Autodesk Fusion 360 part; units mm, degrees
(part 6 of 6)
  spline S39 degree 5 poles (-10.607, 23.738) (-10.6081, 23.7269) (-10.6103, 23.7048) (-10.6136, 23.6717) (-10.6177, 23.6275) (-10.6227, 23.5724) (-10.6274, 23.5173) (-10.6319, 23.4622) (-10.6361, 23.4072) (-10.6401, 23.3523) (-10.6438, 23.2974) (-10.6473, 23.2426) (-10.6505, 23.1878) (-10.6534, 23.133) (-10.6561, 23.0784) (-10.6586, 23.0238) (-10.6607, 22.9692) (-10.6627, 22.9147) (-10.6643, 22.8603) (-10.6657, 22.8059) (-10.6668, 22.7516) (-10.6677, 22.6974) (-10.6683, 22.6432) (-10.6686, 22.5891) (-10.6686, 22.5351) (-10.6684, 22.4812) (-10.6679, 22.4273) (-10.6671, 22.3735) (-10.6661, 22.3198) (-10.6647, 22.2661) (-10.6631, 22.2126) (-10.6612, 22.1591) (-10.659, 22.1057) (-10.6565, 22.0524) (-10.6537, 21.9992) (-10.6506, 21.9461) (-10.6473, 21.893) (-10.6436, 21.8401) (-10.6396, 21.7872) (-10.6353, 21.7345) (-10.6307, 21.6818) (-10.6258, 21.6293) (-10.6205, 21.5768) (-10.615, 21.5245) (-10.6091, 21.4723) (-10.6028, 21.4202) (-10.5963, 21.3682) (-10.5894, 21.3163) (-10.5822, 21.2645) (-10.5746, 21.2129) (-10.5667, 21.1614) (-10.5583, 21.11) (-10.5496, 21.0588) (-10.5405, 21.0078) (-10.531, 20.9569) (-10.5211, 20.9061) (-10.5109, 20.8555) (-10.5003, 20.805) (-10.4893, 20.7546) (-10.4779, 20.7044) (-10.466, 20.6545) (-10.4535, 20.6048) (-10.4404, 20.5553) (-10.4266, 20.5061) (-10.4123, 20.4572) (-10.3976, 20.4084) (-10.3826, 20.3597) (-10.3673, 20.3113) (-10.3516, 20.263) (-10.335, 20.2151) (-10.3172, 20.1677) (-10.3015, 20.1305) (-10.2887, 20.103) (-10.2797, 20.0849) (-10.2751, 20.0759) knots -1 -1 -1 -1 -1 -1 -0.98571429 -0.97142857 -0.95714286 -0.94285714 -0.92857143 -0.91428571 -0.9 -0.88571429 -0.87142857 -0.85714286 -0.84285714 -0.82857143 -0.81428571 -0.8 -0.78571429 -0.77142857 -0.75714286 -0.74285714 -0.72857143 -0.71428571 -0.7 -0.68571429 -0.67142857 -0.65714286 -0.64285714 -0.62857143 -0.61428571 -0.6 -0.58571429 -0.57142857 -0.55714286 -0.54285714 -0.52857143 -0.51428571 -0.5 -0.48571429 -0.47142857 -0.45714286 -0.44285714 -0.42857143 -0.41428571 -0.4 -0.38571429 -0.37142857 -0.35714286 -0.34285714 -0.32857143 -0.31428571 -0.3 -0.28571429 -0.27142857 -0.25714286 -0.24285714 -0.22857143 -0.21428571 -0.2 -0.18571429 -0.17142857 -0.15714286 -0.14285714 -0.12857143 -0.11428571 -0.1 -0.08571429 -0.07142857 -0.05714286 -0.04285714 -0.02857143 -0.01428571 0 0 0 0 0 0
  line L43 (-10.2751, 20.0759) -> (-10.2631, 20.0524)
  arc A79 (-10.659, 18.7284) -> (-10.2631, 20.0524) centre (-11.1537, 19.5975) ccw
  arc A80 (-10.659, 18.7284) -> (-10.8898, 18.5952) centre (0, 0) ccw
  arc A81 (-12.2343, 18.9143) -> (-10.8898, 18.5952) centre (-11.3951, 19.4581) ccw
  line L44 (-12.2343, 18.9143) -> (-12.2487, 18.9365)
  spline S40 degree 5 poles (-12.2487, 18.9365) (-12.2542, 18.945) (-12.2654, 18.9618) (-12.2828, 18.9866) (-12.3072, 19.0188) (-12.3392, 19.0579) (-12.3725, 19.0962) (-12.4064, 19.134) (-12.4407, 19.1715) (-12.4754, 19.2088) (-12.5103, 19.2459) (-12.5455, 19.2828) (-12.5812, 19.3193) (-12.6175, 19.3554) (-12.6543, 19.3911) (-12.6916, 19.4264) (-12.7294, 19.4613) (-12.7675, 19.496) (-12.8059, 19.5304) (-12.8447, 19.5646) (-12.8837, 19.5985) (-12.923, 19.6322) (-12.9627, 19.6656) (-13.0027, 19.6988) (-13.043, 19.7317) (-13.0836, 19.7643) (-13.1245, 19.7967) (-13.1658, 19.8288) (-13.2072, 19.8607) (-13.249, 19.8924) (-13.291, 19.9239) (-13.3333, 19.9551) (-13.3758, 19.9861) (-13.4186, 20.0168) (-13.4616, 20.0474) (-13.5049, 20.0777) (-13.5485, 20.1078) (-13.5923, 20.1376) (-13.6363, 20.1673) (-13.6805, 20.1968) (-13.725, 20.226) (-13.7697, 20.255) (-13.8146, 20.2838) (-13.8597, 20.3124) (-13.9051, 20.3408) (-13.9507, 20.369) (-13.9965, 20.397) (-14.0425, 20.4248) (-14.0887, 20.4523) (-14.1351, 20.4797) (-14.1817, 20.5069) (-14.2285, 20.5339) (-14.2755, 20.5606) (-14.3227, 20.5872) (-14.3701, 20.6136) (-14.4177, 20.6397) (-14.4654, 20.6657) (-14.5134, 20.6915) (-14.5615, 20.7171) (-14.6099, 20.7425) (-14.6584, 20.7676) (-14.7071, 20.7926) (-14.756, 20.8175) (-14.805, 20.8421) (-14.8542, 20.8665) (-14.9036, 20.8907) (-14.9532, 20.9147) (-15.0029, 20.9386) (-15.0529, 20.9622) (-15.1029, 20.9857) (-15.1532, 21.009) (-15.1935, 21.0275) (-15.2238, 21.0412) (-15.2441, 21.0504) (-15.2542, 21.0549) knots 0 0 0 0 0 0 0.01428571 0.02857143 0.04285714 0.05714286 0.07142857 0.08571429 0.1 0.11428571 0.12857143 0.14285714 0.15714286 0.17142857 0.18571429 0.2 0.21428571 0.22857143 0.24285714 0.25714286 0.27142857 0.28571429 0.3 0.31428571 0.32857143 0.34285714 0.35714286 0.37142857 0.38571429 0.4 0.41428571 0.42857143 0.44285714 0.45714286 0.47142857 0.48571429 0.5 0.51428571 0.52857143 0.54285714 0.55714286 0.57142857 0.58571429 0.6 0.61428571 0.62857143 0.64285714 0.65714286 0.67142857 0.68571429 0.7 0.71428571 0.72857143 0.74285714 0.75714286 0.77142857 0.78571429 0.8 0.81428571 0.82857143 0.84285714 0.85714286 0.87142857 0.88571429 0.9 0.91428571 0.92857143 0.94285714 0.95714286 0.97142857 0.98571429 1 1 1 1 1 1
  arc A82 (-15.2542, 21.0549) -> (-16.3894, 20.1838) centre (0, 0) ccw
  spline S41 degree 5 poles (-16.3894, 20.1838) (-16.3876, 20.1729) (-16.384, 20.1509) (-16.3786, 20.1181) (-16.3712, 20.0744) (-16.3617, 20.0198) (-16.352, 19.9654) (-16.3421, 19.911) (-16.3319, 19.8568) (-16.3215, 19.8027) (-16.3109, 19.7487) (-16.3001, 19.6949) (-16.289, 19.6411) (-16.2777, 19.5875) (-16.2661, 19.534) (-16.2544, 19.4806) (-16.2423, 19.4273) (-16.2301, 19.3742) (-16.2176, 19.3212) (-16.2049, 19.2683) (-16.1919, 19.2156) (-16.1787, 19.163) (-16.1653, 19.1105) (-16.1516, 19.0582) (-16.1376, 19.006) (-16.1235, 18.954) (-16.109, 18.9021) (-16.0944, 18.8503) (-16.0794, 18.7987) (-16.0643, 18.7472) (-16.0488, 18.6959) (-16.0331, 18.6447) (-16.0172, 18.5937) (-16.001, 18.5429) (-15.9845, 18.4922) (-15.9678, 18.4417) (-15.9508, 18.3913) (-15.9335, 18.3411) (-15.916, 18.2911) (-15.8982, 18.2413) (-15.8801, 18.1916) (-15.8618, 18.1421) (-15.8431, 18.0928) (-15.8242, 18.0437) (-15.805, 17.9948) (-15.7855, 17.9461) (-15.7657, 17.8976) (-15.7456, 17.8492) (-15.7253, 17.8011) (-15.7046, 17.7532) (-15.6836, 17.7055) (-15.6622, 17.658) (-15.6406, 17.6108) (-15.6185, 17.5639) (-15.5962, 17.5172) (-15.5735, 17.4707) (-15.5505, 17.4244) (-15.5272, 17.3784) (-15.5036, 17.3326) (-15.4796, 17.2871) (-15.4552, 17.2419) (-15.4302, 17.1971) (-15.4048, 17.1527) (-15.3787, 17.1088) (-15.3523, 17.0652) (-15.3254, 17.0219) (-15.2983, 16.9788) (-15.271, 16.9359) (-15.2433, 16.8933) (-15.2149, 16.8513) (-15.1854, 16.8103) (-15.1606, 16.7784) (-15.1412, 16.7551) (-15.1278, 16.74) (-15.121, 16.7325) knots -1 -1 -1 -1 -1 -1 -0.98571429 -0.97142857 -0.95714286 -0.94285714 -0.92857143 -0.91428571 -0.9 -0.88571429 -0.87142857 -0.85714286 -0.84285714 -0.82857143 -0.81428571 -0.8 -0.78571429 -0.77142857 -0.75714286 -0.74285714 -0.72857143 -0.71428571 -0.7 -0.68571429 -0.67142857 -0.65714286 -0.64285714 -0.62857143 -0.61428571 -0.6 -0.58571429 -0.57142857 -0.55714286 -0.54285714 -0.52857143 -0.51428571 -0.5 -0.48571429 -0.47142857 -0.45714286 -0.44285714 -0.42857143 -0.41428571 -0.4 -0.38571429 -0.37142857 -0.35714286 -0.34285714 -0.32857143 -0.31428571 -0.3 -0.28571429 -0.27142857 -0.25714286 -0.24285714 -0.22857143 -0.21428571 -0.2 -0.18571429 -0.17142857 -0.15714286 -0.14285714 -0.12857143 -0.11428571 -0.1 -0.08571429 -0.07142857 -0.05714286 -0.04285714 -0.02857143 -0.01428571 0 0 0 0 0 0
  line L45 (-15.121, 16.7325) -> (-15.1034, 16.7129)
  arc A83 (-15.1431, 15.3315) -> (-15.1034, 16.7129) centre (-15.8458, 16.043) ccw
  arc A84 (-15.1431, 15.3315) -> (-15.3315, 15.1431) centre (0, 0) ccw
  arc A85 (-16.7129, 15.1034) -> (-15.3315, 15.1431) centre (-16.043, 15.8458) ccw
  line L46 (-16.7129, 15.1034) -> (-16.7325, 15.121)
  spline S42 degree 5 poles (-16.7325, 15.121) (-16.74, 15.1278) (-16.7551, 15.1412) (-16.7784, 15.1606) (-16.8103, 15.1854) (-16.8513, 15.2149) (-16.8933, 15.2433) (-16.9359, 15.271) (-16.9788, 15.2983) (-17.0219, 15.3254) (-17.0652, 15.3523) (-17.1088, 15.3787) (-17.1527, 15.4048) (-17.1971, 15.4302) (-17.2419, 15.4552) (-17.2871, 15.4796) (-17.3326, 15.5036) (-17.3784, 15.5272) (-17.4244, 15.5505) (-17.4707, 15.5735) (-17.5172, 15.5962) (-17.5639, 15.6185) (-17.6108, 15.6406) (-17.658, 15.6622) (-17.7055, 15.6836) (-17.7532, 15.7046) (-17.8011, 15.7253) (-17.8492, 15.7456) (-17.8976, 15.7657) (-17.9461, 15.7855) (-17.9948, 15.805) (-18.0437, 15.8242) (-18.0928, 15.8431) (-18.1421, 15.8618) (-18.1916, 15.8801) (-18.2413, 15.8982) (-18.2911, 15.916) (-18.3411, 15.9335) (-18.3913, 15.9508) (-18.4417, 15.9678) (-18.4922, 15.9845) (-18.5429, 16.001) (-18.5937, 16.0172) (-18.6447, 16.0331) (-18.6959, 16.0488) (-18.7472, 16.0643) (-18.7987, 16.0794) (-18.8503, 16.0944) (-18.9021, 16.109) (-18.954, 16.1235) (-19.006, 16.1376) (-19.0582, 16.1516) (-19.1105, 16.1653) (-19.163, 16.1787) (-19.2156, 16.1919) (-19.2683, 16.2049) (-19.3212, 16.2176) (-19.3742, 16.2301) (-19.4273, 16.2423) (-19.4806, 16.2544) (-19.534, 16.2661) (-19.5875, 16.2777) (-19.6411, 16.289) (-19.6949, 16.3001) (-19.7487, 16.3109) (-19.8027, 16.3215) (-19.8568, 16.3319) (-19.911, 16.3421) (-19.9654, 16.352) (-20.0198, 16.3617) (-20.0744, 16.3712) (-20.1181, 16.3786) (-20.1509, 16.384) (-20.1729, 16.3876) (-20.1838, 16.3894) knots 0 0 0 0 0 0 0.01428571 0.02857143 0.04285714 0.05714286 0.07142857 0.08571429 0.1 0.11428571 0.12857143 0.14285714 0.15714286 0.17142857 0.18571429 0.2 0.21428571 0.22857143 0.24285714 0.25714286 0.27142857 0.28571429 0.3 0.31428571 0.32857143 0.34285714 0.35714286 0.37142857 0.38571429 0.4 0.41428571 0.42857143 0.44285714 0.45714286 0.47142857 0.48571429 0.5 0.51428571 0.52857143 0.54285714 0.55714286 0.57142857 0.58571429 0.6 0.61428571 0.62857143 0.64285714 0.65714286 0.67142857 0.68571429 0.7 0.71428571 0.72857143 0.74285714 0.75714286 0.77142857 0.78571429 0.8 0.81428571 0.82857143 0.84285714 0.85714286 0.87142857 0.88571429 0.9 0.91428571 0.92857143 0.94285714 0.95714286 0.97142857 0.98571429 1 1 1 1 1 1
  arc A86 (-20.1838, 16.3894) -> (-21.0549, 15.2542) centre (0, 0) ccw
  spline S43 degree 5 poles (-21.0549, 15.2542) (-21.0504, 15.2441) (-21.0412, 15.2238) (-21.0275, 15.1935) (-21.009, 15.1532) (-20.9857, 15.1029) (-20.9622, 15.0529) (-20.9386, 15.0029) (-20.9147, 14.9532) (-20.8907, 14.9036) (-20.8665, 14.8542) (-20.8421, 14.805) (-20.8175, 14.756) (-20.7926, 14.7071) (-20.7676, 14.6584) (-20.7425, 14.6099) (-20.7171, 14.5615) (-20.6915, 14.5134) (-20.6657, 14.4654) (-20.6397, 14.4177) (-20.6136, 14.3701) (-20.5872, 14.3227) (-20.5606, 14.2755) (-20.5339, 14.2285) (-20.5069, 14.1817) (-20.4797, 14.1351) (-20.4523, 14.0887) (-20.4248, 14.0425) (-20.397, 13.9965) (-20.369, 13.9507) (-20.3408, 13.9051) (-20.3124, 13.8597) (-20.2838, 13.8146) (-20.255, 13.7697) (-20.226, 13.725) (-20.1968, 13.6805) (-20.1673, 13.6363) (-20.1376, 13.5923) (-20.1078, 13.5485) (-20.0777, 13.5049) (-20.0474, 13.4616) (-20.0168, 13.4186) (-19.9861, 13.3758) (-19.9551, 13.3333) (-19.9239, 13.291) (-19.8924, 13.249) (-19.8607, 13.2072) (-19.8288, 13.1658) (-19.7967, 13.1245) (-19.7643, 13.0836) (-19.7317, 13.043) (-19.6988, 13.0027) (-19.6656, 12.9627) (-19.6322, 12.923) (-19.5985, 12.8837) (-19.5646, 12.8447) (-19.5304, 12.8059) (-19.496, 12.7675) (-19.4613, 12.7294) (-19.4264, 12.6916) (-19.3911, 12.6543) (-19.3554, 12.6175) (-19.3193, 12.5812) (-19.2828, 12.5455) (-19.2459, 12.5103) (-19.2088, 12.4754) (-19.1715, 12.4407) (-19.134, 12.4064) (-19.0962, 12.3725) (-19.0579, 12.3392) (-19.0188, 12.3072) (-18.9866, 12.2828) (-18.9618, 12.2654) (-18.945, 12.2542) (-18.9365, 12.2487) knots -1 -1 -1 -1 -1 -1 -0.98571429 -0.97142857 -0.95714286 -0.94285714 -0.92857143 -0.91428571 -0.9 -0.88571429 -0.87142857 -0.85714286 -0.84285714 -0.82857143 -0.81428571 -0.8 -0.78571429 -0.77142857 -0.75714286 -0.74285714 -0.72857143 -0.71428571 -0.7 -0.68571429 -0.67142857 -0.65714286 -0.64285714 -0.62857143 -0.61428571 -0.6 -0.58571429 -0.57142857 -0.55714286 -0.54285714 -0.52857143 -0.51428571 -0.5 -0.48571429 -0.47142857 -0.45714286 -0.44285714 -0.42857143 -0.41428571 -0.4 -0.38571429 -0.37142857 -0.35714286 -0.34285714 -0.32857143 -0.31428571 -0.3 -0.28571429 -0.27142857 -0.25714286 -0.24285714 -0.22857143 -0.21428571 -0.2 -0.18571429 -0.17142857 -0.15714286 -0.14285714 -0.12857143 -0.11428571 -0.1 -0.08571429 -0.07142857 -0.05714286 -0.04285714 -0.02857143 -0.01428571 0 0 0 0 0 0
  line L47 (-18.9365, 12.2487) -> (-18.9143, 12.2343)
  arc A87 (-18.5952, 10.8898) -> (-18.9143, 12.2343) centre (-19.4581, 11.3951) ccw
  arc A88 (-18.5952, 10.8898) -> (-18.7284, 10.659) centre (0, 0) ccw
  arc A89 (-20.0524, 10.2631) -> (-18.7284, 10.659) centre (-19.5975, 11.1537) ccw
  line L48 (-20.0524, 10.2631) -> (-20.0759, 10.2751)
  spline S44 degree 5 poles (-20.0759, 10.2751) (-20.0849, 10.2797) (-20.103, 10.2887) (-20.1305, 10.3015) (-20.1677, 10.3172) (-20.2151, 10.335) (-20.263, 10.3516) (-20.3113, 10.3673) (-20.3597, 10.3826) (-20.4084, 10.3976) (-20.4572, 10.4123) (-20.5061, 10.4266) (-20.5553, 10.4404) (-20.6048, 10.4535) (-20.6545, 10.466) (-20.7044, 10.4779) (-20.7546, 10.4893) (-20.805, 10.5003) (-20.8555, 10.5109) (-20.9061, 10.5211) (-20.9569, 10.531) (-21.0078, 10.5405) (-21.0588, 10.5496) (-21.11, 10.5583) (-21.1614, 10.5667) (-21.2129, 10.5746) (-21.2645, 10.5822) (-21.3163, 10.5894) (-21.3682, 10.5963) (-21.4202, 10.6028) (-21.4723, 10.6091) (-21.5245, 10.615) (-21.5768, 10.6205) (-21.6293, 10.6258) (-21.6818, 10.6307) (-21.7345, 10.6353) (-21.7872, 10.6396) (-21.8401, 10.6436) (-21.893, 10.6473) (-21.9461, 10.6506) (-21.9992, 10.6537) (-22.0524, 10.6565) (-22.1057, 10.659) (-22.1591, 10.6612) (-22.2126, 10.6631) (-22.2661, 10.6647) (-22.3198, 10.6661) (-22.3735, 10.6671) (-22.4273, 10.6679) (-22.4812, 10.6684) (-22.5351, 10.6686) (-22.5891, 10.6686) (-22.6432, 10.6683) (-22.6974, 10.6677) (-22.7516, 10.6668) (-22.8059, 10.6657) (-22.8603, 10.6643) (-22.9147, 10.6627) (-22.9692, 10.6607) (-23.0238, 10.6586) (-23.0784, 10.6561) (-23.133, 10.6534) (-23.1878, 10.6505) (-23.2426, 10.6473) (-23.2974, 10.6438) (-23.3523, 10.6401) (-23.4072, 10.6361) (-23.4622, 10.6319) (-23.5173, 10.6274) (-23.5724, 10.6227) (-23.6275, 10.6177) (-23.6717, 10.6136) (-23.7048, 10.6103) (-23.7269, 10.6081) (-23.738, 10.607) knots 0 0 0 0 0 0 0.01428571 0.02857143 0.04285714 0.05714286 0.07142857 0.08571429 0.1 0.11428571 0.12857143 0.14285714 0.15714286 0.17142857 0.18571429 0.2 0.21428571 0.22857143 0.24285714 0.25714286 0.27142857 0.28571429 0.3 0.31428571 0.32857143 0.34285714 0.35714286 0.37142857 0.38571429 0.4 0.41428571 0.42857143 0.44285714 0.45714286 0.47142857 0.48571429 0.5 0.51428571 0.52857143 0.54285714 0.55714286 0.57142857 0.58571429 0.6 0.61428571 0.62857143 0.64285714 0.65714286 0.67142857 0.68571429 0.7 0.71428571 0.72857143 0.74285714 0.75714286 0.77142857 0.78571429 0.8 0.81428571 0.82857143 0.84285714 0.85714286 0.87142857 0.88571429 0.9 0.91428571 0.92857143 0.94285714 0.95714286 0.97142857 0.98571429 1 1 1 1 1 1
  arc A90 (-23.738, 10.607) -> (-24.2856, 9.285) centre (0, 0) ccw
  spline S45 degree 5 poles (-24.2856, 9.285) (-24.2785, 9.2764) (-24.2645, 9.2592) (-24.2433, 9.2335) (-24.2151, 9.1993) (-24.1796, 9.1568) (-24.1439, 9.1145) (-24.1082, 9.0724) (-24.0723, 9.0306) (-24.0362, 8.9889) (-24, 8.9474) (-23.9637, 8.9062) (-23.9272, 8.8652) (-23.8906, 8.8244) (-23.8539, 8.7839) (-23.817, 8.7435) (-23.78, 8.7034) (-23.7428, 8.6635) (-23.7055, 8.6239) (-23.668, 8.5844) (-23.6304, 8.5452) (-23.5927, 8.5063) (-23.5548, 8.4676) (-23.5168, 8.4291) (-23.4786, 8.3909) (-23.4403, 8.3529) (-23.4019, 8.3151) (-23.3633, 8.2777) (-23.3245, 8.2404) (-23.2857, 8.2034) (-23.2466, 8.1667) (-23.2075, 8.1302) (-23.1682, 8.094) (-23.1287, 8.0581) (-23.0891, 8.0225) (-23.0493, 7.9871) (-23.0095, 7.9519) (-22.9694, 7.9171) (-22.9292, 7.8826) (-22.8889, 7.8483) (-22.8484, 7.8143) (-22.8078, 7.7806) (-22.767, 7.7473) (-22.726, 7.7142) (-22.6849, 7.6815) (-22.6437, 7.649) (-22.6023, 7.6169) (-22.5607, 7.5851) (-22.519, 7.5536) (-22.4772, 7.5224) (-22.4351, 7.4916) (-22.3929, 7.4612) (-22.3505, 7.4311) (-22.308, 7.4015) (-22.2653, 7.3722) (-22.2224, 7.3433) (-22.1793, 7.3147) (-22.1361, 7.2865) (-22.0928, 7.2587) (-22.0493, 7.2312) (-22.0055, 7.2043) (-21.9615, 7.178) (-21.9173, 7.1523) (-21.8728, 7.1273) (-21.828, 7.1028) (-21.7832, 7.0787) (-21.7381, 7.0549) (-21.693, 7.0314) (-21.6478, 7.0084) (-21.6022, 6.9862) (-21.5561, 6.9654) (-21.5187, 6.9502) (-21.4902, 6.9398) (-21.471, 6.9333) (-21.4614, 6.9302) knots -1 -1 -1 -1 -1 -1 -0.98571429 -0.97142857 -0.95714286 -0.94285714 -0.92857143 -0.91428571 -0.9 -0.88571429 -0.87142857 -0.85714286 -0.84285714 -0.82857143 -0.81428571 -0.8 -0.78571429 -0.77142857 -0.75714286 -0.74285714 -0.72857143 -0.71428571 -0.7 -0.68571429 -0.67142857 -0.65714286 -0.64285714 -0.62857143 -0.61428571 -0.6 -0.58571429 -0.57142857 -0.55714286 -0.54285714 -0.52857143 -0.51428571 -0.5 -0.48571429 -0.47142857 -0.45714286 -0.44285714 -0.42857143 -0.41428571 -0.4 -0.38571429 -0.37142857 -0.35714286 -0.34285714 -0.32857143 -0.31428571 -0.3 -0.28571429 -0.27142857 -0.25714286 -0.24285714 -0.22857143 -0.21428571 -0.2 -0.18571429 -0.17142857 -0.15714286 -0.14285714 -0.12857143 -0.11428571 -0.1 -0.08571429 -0.07142857 -0.05714286 -0.04285714 -0.02857143 -0.01428571 0 0 0 0 0 0
  line L49 (-21.4614, 6.9302) -> (-21.4363, 6.9221)
  arc A91 (-20.78, 5.7059) -> (-21.4363, 6.9221) centre (-21.7444, 5.9707) ccw
  arc A92 (-20.78, 5.7059) -> (-20.849, 5.4485) centre (0, 0) ccw
  arc A93 (-22.0254, 4.7235) -> (-20.849, 5.4485) centre (-21.8165, 5.7014) ccw
  line L50 (-22.0254, 4.7235) -> (-22.0512, 4.729)
  spline S46 degree 5 poles (-22.0512, 4.729) (-22.0611, 4.7311) (-22.081, 4.7351) (-22.1108, 4.7403) (-22.1508, 4.7458) (-22.2011, 4.7508) (-22.2517, 4.7544) (-22.3024, 4.7571) (-22.3532, 4.7594) (-22.4041, 4.7613) (-22.455, 4.7629) (-22.506, 4.764) (-22.5571, 4.7645) (-22.6082, 4.7644) (-22.6595, 4.7636) (-22.7108, 4.7622) (-22.7623, 4.7602) (-22.8137, 4.7578) (-22.8652, 4.7549) (-22.9168, 4.7517) (-22.9684, 4.7481) (-23.02, 4.7441) (-23.0717, 4.7397) (-23.1234, 4.7349) (-23.1752, 4.7296) (-23.227, 4.724) (-23.2788, 4.7179) (-23.3307, 4.7115) (-23.3826, 4.7047) (-23.4345, 4.6976) (-23.4865, 4.6901) (-23.5384, 4.6823) (-23.5904, 4.6742) (-23.6424, 4.6656) (-23.6945, 4.6568) (-23.7465, 4.6476) (-23.7986, 4.6381) (-23.8506, 4.6283) (-23.9027, 4.6181) (-23.9548, 4.6077) (-24.007, 4.5969) (-24.0591, 4.5858) (-24.1112, 4.5744) (-24.1634, 4.5627) (-24.2155, 4.5507) (-24.2677, 4.5384) (-24.3198, 4.5259) (-24.372, 4.513) (-24.4242, 4.4998) (-24.4763, 4.4863) (-24.5285, 4.4726) (-24.5807, 4.4586) (-24.6328, 4.4443) (-24.685, 4.4297) (-24.7372, 4.4148) (-24.7893, 4.3997) (-24.8415, 4.3843) (-24.8936, 4.3686) (-24.9458, 4.3526) (-24.9979, 4.3364) (-25.05, 4.3199) (-25.1021, 4.3031) (-25.1542, 4.2861) (-25.2063, 4.2688) (-25.2584, 4.2513) (-25.3104, 4.2335) (-25.3625, 4.2154) (-25.4145, 4.1971) (-25.4665, 4.1786) (-25.5185, 4.1598) (-25.5705, 4.1407) (-25.6121, 4.1252) (-25.6433, 4.1135) (-25.664, 4.1057) (-25.6744, 4.1017) knots 0 0 0 0 0 0 0.01428571 0.02857143 0.04285714 0.05714286 0.07142857 0.08571429 0.1 0.11428571 0.12857143 0.14285714 0.15714286 0.17142857 0.18571429 0.2 0.21428571 0.22857143 0.24285714 0.25714286 0.27142857 0.28571429 0.3 0.31428571 0.32857143 0.34285714 0.35714286 0.37142857 0.38571429 0.4 0.41428571 0.42857143 0.44285714 0.45714286 0.47142857 0.48571429 0.5 0.51428571 0.52857143 0.54285714 0.55714286 0.57142857 0.58571429 0.6 0.61428571 0.62857143 0.64285714 0.65714286 0.67142857 0.68571429 0.7 0.71428571 0.72857143 0.74285714 0.75714286 0.77142857 0.78571429 0.8 0.81428571 0.82857143 0.84285714 0.85714286 0.87142857 0.88571429 0.9 0.91428571 0.92857143 0.94285714 0.95714286 0.97142857 0.98571429 1 1 1 1 1 1
  arc A94 (-25.6744, 4.1017) -> (-25.8612, 2.6831) centre (0, 0) ccw
  spline S47 degree 5 poles (-25.8612, 2.6831) (-25.8522, 2.6766) (-25.8341, 2.6636) (-25.8071, 2.6442) (-25.7709, 2.6185) (-25.7256, 2.5867) (-25.6803, 2.555) (-25.6348, 2.5236) (-25.5893, 2.4925) (-25.5437, 2.4616) (-25.498, 2.4309) (-25.4523, 2.4005) (-25.4064, 2.3703) (-25.3605, 2.3404) (-25.3145, 2.3107) (-25.2684, 2.2813) (-25.2223, 2.2521) (-25.1761, 2.2232) (-25.1297, 2.1946) (-25.0834, 2.1662) (-25.0369, 2.1381) (-24.9904, 2.1102) (-24.9438, 2.0826) (-24.8971, 2.0553) (-24.8503, 2.0282) (-24.8035, 2.0015) (-24.7566, 1.975) (-24.7096, 1.9487) (-24.6625, 1.9228) (-24.6154, 1.8971) (-24.5682, 1.8718) (-24.521, 1.8467) (-24.4736, 1.8219) (-24.4262, 1.7974) (-24.3787, 1.7732) (-24.3312, 1.7493) (-24.2835, 1.7257) (-24.2358, 1.7024) (-24.1881, 1.6794) (-24.1403, 1.6568) (-24.0924, 1.6344) (-24.0444, 1.6124) (-23.9963, 1.5908) (-23.9482, 1.5694) (-23.9001, 1.5484) (-23.8518, 1.5278) (-23.8035, 1.5075) (-23.7551, 1.4875) (-23.7067, 1.4678) (-23.6582, 1.4486) (-23.6096, 1.4297) (-23.561, 1.4112) (-23.5123, 1.3932) (-23.4635, 1.3756) (-23.4147, 1.3583) (-23.3658, 1.3415) (-23.3168, 1.3251) (-23.2678, 1.309) (-23.2187, 1.2933) (-23.1695, 1.2781) (-23.1203, 1.2634) (-23.071, 1.2494) (-23.0216, 1.236) (-22.9721, 1.2233) (-22.9226, 1.2112) (-22.873, 1.1996) (-22.8234, 1.1882) (-22.7737, 1.1773) (-22.724, 1.1668) (-22.6743, 1.1571) (-22.6244, 1.1489) (-22.5843, 1.1439) (-22.5541, 1.1413) (-22.5339, 1.14) (-22.5238, 1.1394) knots -1 -1 -1 -1 -1 -1 -0.98571429 -0.97142857 -0.95714286 -0.94285714 -0.92857143 -0.91428571 -0.9 -0.88571429 -0.87142857 -0.85714286 -0.84285714 -0.82857143 -0.81428571 -0.8 -0.78571429 -0.77142857 -0.75714286 -0.74285714 -0.72857143 -0.71428571 -0.7 -0.68571429 -0.67142857 -0.65714286 -0.64285714 -0.62857143 -0.61428571 -0.6 -0.58571429 -0.57142857 -0.55714286 -0.54285714 -0.52857143 -0.51428571 -0.5 -0.48571429 -0.47142857 -0.45714286 -0.44285714 -0.42857143 -0.41428571 -0.4 -0.38571429 -0.37142857 -0.35714286 -0.34285714 -0.32857143 -0.31428571 -0.3 -0.28571429 -0.27142857 -0.25714286 -0.24285714 -0.22857143 -0.21428571 -0.2 -0.18571429 -0.17142857 -0.15714286 -0.14285714 -0.12857143 -0.11428571 -0.1 -0.08571429 -0.07142857 -0.05714286 -0.04285714 -0.02857143 -0.01428571 0 0 0 0 0 0
  line L51 (-22.5238, 1.1394) -> (-22.4975, 1.1381)
  arc A95 (-21.5488, 0.1332) -> (-22.4975, 1.1381) centre (-22.5488, 0.1394) ccw
  circle A96 centre (0, 0) radius 6.35
  line L52 (-70, 15) -> (-24.9077, -25.8612)
  constraint coincident L1 L52.start
  constraint coincident L2 L52.end
sketch "スケッチ2 (4)" plane through (0, 0, 0) normal (0, 0, 1) x (-1, 0, 0)
  line L0 (80, 29.8124) -> (-70, 29.8124)
  line L1 (-70, 29.8124) -> (-70, -25.8612)
  line L2 (-70, -25.8612) -> (80, -25.8612)
  line L3 (80, -25.8612) -> (80, 29.8124)
sketch "スケッチ3 (3)" plane through (0, 0, -2) normal (0, 0, -1) x (1, 0, 0)
  line L0 (-80, -25.8612) -> (70, -25.8612)
  line L1 (70, -25.8612) -> (70, 29.8124)
  line L2 (70, 29.8124) -> (-80, 29.8124)
  line L3 (-80, 29.8124) -> (-80, -25.8612)
  circle A0 centre (0, 0) radius 16
  dimension "d32" = 32
  constraint coincident A0.centre origin
  measures "d32" diameter of A0
sketch "スケッチ4" plane through (0, 0, -2) normal (0, 0, -1) x (1, 0, 0)
  line L0 (-80, -25.8612) -> (70, -25.8612)
  line L1 (70, -25.8612) -> (70, 29.8124)
  line L2 (70, 29.8124) -> (-80, 29.8124)
  line L3 (-80, 29.8124) -> (-80, -25.8612)
  circle A0 centre (0, 0) radius 16
  circle A1 centre (0, 0) radius 6.2
  dimension "d35" = 12.4
  constraint coincident A0.centre A1.centre
  measures "d35" diameter of A1
extrude "押し出し3" cut sketch "スケッチ3 (3)" against normal blind 1 contours A0 bodies 24 in component "Base1"
extrude "押し出し4" cut sketch "スケッチ4" against normal blind 17 contours A1 bodies 24 in component "Base1"
sketch "スケッチ5" plane through (0, 0, -1) normal (0, 0, -1) x (1, 0, 0)
  circle A0 centre (0, 0) radius 6.2
  circle A1 centre (0, 0) radius 16
  circle A2 centre (0, 0) radius 6.35
  circle A3 centre (0, 0) radius 16
  line L0 (0, -25.8612) -> (0, 29.8124)
  circle A4 centre (0, 0) radius 6
  dimension "d38" = 12
  constraint coincident A0.centre A1.centre
  measures "d38" diameter of A4
extrude "押し出し1'''" add sketch "スケッチ5" against normal blind 15 separate body contours L0 A4 | L0 A4 makes body 25
sketch "スケッチ6" plane through (0, 0, -1) normal (0, 0, -1) x (1, 0, 0)
  circle A0 centre (0, 0) radius 6
  circle A1 centre (0, 0) radius 15.65
  dimension "d43" = 31.3
  constraint concentric A0 A1
  measures "d43" diameter of A1
extrude "押し出し2'''" add sketch "スケッチ5" sketch "スケッチ6" along normal blind 1 contours L0 A4 | L0 A4 of sketch 2 bodies 25
component "Spur Gear (24 teeth)" placed x (1, 0, 0) y (0, 1, 0) z (0, 0, 1) at (0, 0, 0)
component "Rack" placed x (1, 0, 0) y (0, 1, 0) z (0, 0, 1) at (0, 0, 0)
component "Base1" placed x (1, 0, 0) y (0, 1, 0) z (0, 0, 1) at (0, 0, 0)
equation "d12 = ( ( 360 / 24 ) / 2 ) * 1 deg"
equation "d17 = ( ( 48 * PI ) / 24 ) * 1 mm"
